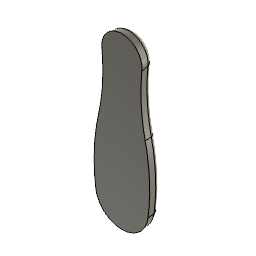
link2 (Autodesk Fusion 360 design; units mm, degrees)
part number: 2025-12-13-22-35-12-355
Autodesk Fusion 360 part; units mm, degrees
sketch "Sketch1" plane through (0, 0, 0) normal (0, 1, 0) x (1, 0, 0)
  arc A0 (35.2531, -100) -> (29.8304, -196.8149) centre (328.1348, -164.9639) ccw
  arc A1 (35.2531, -100) -> (39.6352, 5.3902) centre (-257.6286, -35.0361) ccw
  line L0 (0, -200) -> (0, 0) construction
  arc A2 (-29.8304, -196.8149) -> (-35.2531, -100) centre (-328.1348, -164.9639) ccw
  arc A3 (-39.6352, 5.3902) -> (-35.2531, -100) centre (257.6286, -35.0361) ccw
  arc A4 (-29.8304, -196.8149) -> (29.8304, -196.8149) centre (0, -200) ccw
  arc A5 (39.6352, 5.3902) -> (-39.6352, 5.3902) centre (0, 0) ccw
  dimension "d1" = 80
  dimension "d2" = 60
  dimension "d3" = 200
  dimension "d7" = 100
  dimension "d8" = 300
  constraint coincident L0.end A5.centre
  constraint vertical L0.end L0.start
  constraint tangent A0 A4
  constraint tangent A0 A1
  constraint tangent A1 A5
  constraint coincident L0.start A4.centre
  constraint symmetric A0.end L0 A2.start
  constraint symmetric A0.start L0 A2.end
  constraint symmetric A0 L0 A2
  constraint symmetric A1.end L0 A3.start
  constraint symmetric A1 L0 A3
  constraint equal A0 A1
  measures "d1" diameter of A5
  measures "d2" diameter of A4
  measures "d3" distance of L0.end L0.start
  measures "d7" vertical distance of L0.end A0.start
  measures "d8" radius of A0
extrude "Extrude1" add sketch "Sketch1" against normal blind 20 draft 8
fillet "Fillet1" radius 10 6 edges at (0, 0, 230) (-28.6043, 0, 148.1869) (-42.1125, 0, 47.499) (0, 0, -40) (42.1125, 0, 47.499) (28.6043, 0, 148.1869)
